Autodesk Inventor part; units mm, degrees
(part 2 of 2)
sketch "Boceto13" plane through (0, 0, 0) normal (0, 0, -1) x (-1, 0, 0)
  circle A0 centre (-56.75, 72.0206) radius 8 projected
  line L0 (-56.75, 72.0206) -> (-80.75, 72.0206)
  line L1 (-80.75, 105.95) -> (-80.75, -105.95) projected
  line L2 (-80.75, 72.0206) -> (80.75, 72.0206)
  line L3 (80.75, -105.95) -> (80.75, 105.95) projected
  circle A1 centre (-56.75, 43.1636) radius 8 projected
  line L4 (-56.75, 43.1636) -> (-56.75, 72.0206)
  line L5 (-56.75, 43.1636) -> (-80.75, 43.1636)
  line L6 (-80.75, 43.1636) -> (80.75, 43.1636)
  line L7 (-56.75, 14.3066) -> (-56.75, 43.1636)
  line L8 (-56.75, 14.3066) -> (-80.75, 14.3066)
  line L9 (-80.75, 14.3066) -> (80.75, 14.3066)
  line L10 (-56.75, -14.5504) -> (-56.75, 14.3066)
  line L11 (-56.75, -14.5504) -> (-80.75, -14.5504)
  line L12 (-80.75, -14.5504) -> (80.75, -14.5504)
  line L13 (-56.75, -43.4074) -> (-56.75, -14.5504)
  line L14 (-56.75, -43.4074) -> (-80.75, -43.4074)
  line L15 (-80.75, -43.4074) -> (80.75, -43.4074)
  line L16 (-56.75, -72.2644) -> (-56.75, -43.4074)
  line L17 (-56.75, -98.6167) -> (-56.75, -69.7597)
  line L18 (-56.75, -72.2644) -> (-80.75, -72.2644)
  line L19 (-80.75, -72.2644) -> (80.75, -72.2644)
  line L20 (-56.75, -101.1214) -> (-56.75, -72.2644)
  line L21 (43.5, 62.1456) -> (30.5, 62.1456) projected
  line L22 (30.5, 62.1456) -> (-80.75, 62.1456)
  line L23 (30.5, 81.8956) -> (43.5, 81.8956) projected
  line L24 (30.5, 81.8956) -> (80.75, 81.8956)
  line L25 (30.5, 62.1456) -> (80.75, 62.1456)
  line L26 (30.5, 81.8956) -> (-80.75, 81.8956)
  line L27 (30.5, 33.2886) -> (-80.75, 33.2886)
  line L28 (30.5, 53.0386) -> (80.75, 53.0386)
  line L29 (30.5, 33.2886) -> (80.75, 33.2886)
  line L30 (30.5, 53.0386) -> (-80.75, 53.0386)
  line L31 (30.5, 4.4316) -> (-80.75, 4.4316)
  line L32 (30.5, 24.1816) -> (80.75, 24.1816)
  line L33 (30.5, 4.4316) -> (80.75, 4.4316)
  line L34 (30.5, 24.1816) -> (-80.75, 24.1816)
  line L35 (30.5, -24.4254) -> (-80.75, -24.4254)
  line L36 (30.5, -4.6754) -> (80.75, -4.6754)
  line L37 (30.5, -24.4254) -> (80.75, -24.4254)
  line L38 (30.5, -4.6754) -> (-80.75, -4.6754)
  line L39 (30.5, -53.2824) -> (-80.75, -53.2824)
  line L40 (30.5, -33.5324) -> (80.75, -33.5324)
  line L41 (30.5, -53.2824) -> (80.75, -53.2824)
  line L42 (30.5, -33.5324) -> (-80.75, -33.5324)
  line L43 (30.5, -82.1394) -> (-80.75, -82.1394)
  line L44 (30.5, -62.3894) -> (80.75, -62.3894)
  line L45 (30.5, -82.1394) -> (80.75, -82.1394)
  line L46 (30.5, -62.3894) -> (-80.75, -62.3894)
  line L47 (-80.6263, 81.8524) -> (-64.7122, 81.8524) construction
  line L48 (-64.7122, 81.8524) -> (-64.7122, 62.1807) construction
  line L49 (-64.7122, 62.1807) -> (-80.6263, 62.1807) construction
  line L50 (-80.6263, 62.1807) -> (-80.6263, 81.8524) construction
  line L51 (-83, 108.2) -> (83, 108.2) projected
  line L52 (0, 108.2) -> (0, -109.1206)
  line L53 (-80.6263, 52.9954) -> (-64.7122, 52.9954) construction
  line L54 (-64.7122, 52.9954) -> (-64.7122, 33.3237) construction
  line L55 (-64.7122, 33.3237) -> (-80.6263, 33.3237) construction
  line L56 (-80.6263, 33.3237) -> (-80.6263, 52.9954) construction
  line L57 (-80.6263, 24.1384) -> (-64.7122, 24.1384) construction
  line L58 (-64.7122, 24.1384) -> (-64.7122, 4.4667) construction
  line L59 (-64.7122, 4.4667) -> (-80.6263, 4.4667) construction
  line L60 (-80.6263, 4.4667) -> (-80.6263, 24.1384) construction
  line L61 (-80.6263, -4.7186) -> (-64.7122, -4.7186) construction
  line L62 (-64.7122, -4.7186) -> (-64.7122, -24.3903) construction
  line L63 (-64.7122, -24.3903) -> (-80.6263, -24.3903) construction
  line L64 (-80.6263, -24.3903) -> (-80.6263, -4.7186) construction
  line L65 (-80.6263, -33.5756) -> (-64.7122, -33.5756) construction
  line L66 (-64.7122, -33.5756) -> (-64.7122, -53.2473) construction
  line L67 (-64.7122, -53.2473) -> (-80.6263, -53.2473) construction
  line L68 (-80.6263, -53.2473) -> (-80.6263, -33.5756) construction
  line L69 (-80.6263, -62.4326) -> (-64.7122, -62.4326) construction
  line L70 (-64.7122, -62.4326) -> (-64.7122, -82.1043) construction
  line L71 (-64.7122, -82.1043) -> (-80.6263, -82.1043) construction
  line L72 (-80.6263, -82.1043) -> (-80.6263, -62.4326) construction
  line L73 (-72.6693, 72.0206) -> (-88.5883, 72.0206)
  circle A2 centre (56.75, 72.0206) radius 8 projected
  circle A3 centre (56.75, -72.2644) radius 8 projected
  line L74 (56.75, 72.0206) -> (56.75, -72.2644)
  line L75 (64.7119, 81.8524) -> (80.6261, 81.8524) construction
  line L76 (80.6261, 81.8524) -> (80.6261, 62.1807) construction
  line L77 (80.6261, 62.1807) -> (64.7119, 62.1807) construction
  line L78 (64.7119, 62.1807) -> (64.7119, 81.8524) construction
  line L79 (56.75, 43.1636) -> (56.75, 14.3066)
  line L80 (56.75, -14.5504) -> (56.75, 14.3066)
  circle A4 centre (56.75, -43.4074) radius 8 projected
  line L81 (56.75, -72.2644) -> (56.75, -43.4074)
  line L82 (56.75, -43.4074) -> (56.75, -14.5504)
  line L83 (64.7119, 33.3237) -> (64.7119, 52.9954) construction
  line L84 (64.7119, 52.9954) -> (80.6261, 52.9954) construction
  line L85 (80.6261, 52.9954) -> (80.6261, 33.3237) construction
  line L86 (80.6261, 33.3237) -> (64.7119, 33.3237) construction
  line L87 (64.7119, 4.4667) -> (64.7119, 24.1384) construction
  line L88 (64.7119, 24.1384) -> (80.6261, 24.1384) construction
  line L89 (80.6261, 24.1384) -> (80.6261, 4.4667) construction
  line L90 (80.6261, 4.4667) -> (64.7119, 4.4667) construction
  line L91 (64.7119, -24.3903) -> (64.7119, -4.7186) construction
  line L92 (64.7119, -4.7186) -> (80.6261, -4.7186) construction
  line L93 (80.6261, -4.7186) -> (80.6261, -24.3903) construction
  line L94 (80.6261, -24.3903) -> (64.7119, -24.3903) construction
  line L95 (64.7119, -53.2473) -> (64.7119, -33.5756) construction
  line L96 (64.7119, -33.5756) -> (80.6261, -33.5756) construction
  line L97 (80.6261, -33.5756) -> (80.6261, -53.2473) construction
  line L98 (80.6261, -53.2473) -> (64.7119, -53.2473) construction
  line L99 (64.7119, -82.1043) -> (64.7119, -62.4326) construction
  line L100 (64.7119, -62.4326) -> (80.6261, -62.4326) construction
  line L101 (80.6261, -62.4326) -> (80.6261, -82.1043) construction
  line L102 (80.6261, -82.1043) -> (64.7119, -82.1043) construction
  spline S0 degree 2 poles (-73.0647, 70.8153) (-73.0647, 70.3655) (-73.3959, 69.629) (-73.7173, 69.3719) knots 0 0 0 1 2 2 2
  spline S1 degree 2 poles (-73.7173, 69.3719) (-74.0386, 69.1149) (-74.9135, 68.838) (-75.5413, 68.838) knots 0 0 0 1 2 2 2
  spline S2 degree 2 poles (-75.5413, 68.838) (-76.2532, 68.838) (-77.2715, 69.0753) (-77.5928, 69.2236) knots 0 0 0 1 2 2 2
  line L103 (-77.5928, 69.2236) -> (-77.5928, 70.5484)
  line L104 (-77.5928, 70.5484) -> (-77.4445, 70.5484)
  spline S3 degree 2 poles (-77.4445, 70.5484) (-77.1083, 70.3358) (-76.2037, 70.0195) (-75.828, 70.0195) knots 0 0 0 1 2 2 2
  spline S4 degree 2 poles (-75.828, 70.0195) (-75.6056, 70.0195) (-75.0865, 70.0986) (-74.9086, 70.2271) knots 0 0 0 1 2 2 2
  spline S5 degree 2 poles (-74.9086, 70.2271) (-74.7702, 70.3309) (-74.6021, 70.6324) (-74.6021, 70.9043) knots 0 0 0 1 2 2 2
  spline S6 degree 2 poles (-74.6021, 70.9043) (-74.6021, 71.1762) (-74.8394, 71.4679) (-75.0371, 71.5371) knots 0 0 0 1 2 2 2
  spline S7 degree 2 poles (-75.0371, 71.5371) (-75.2348, 71.6063) (-75.7835, 71.6211) (-75.9961, 71.6211) knots 0 0 0 1 2 2 2
  line L105 (-75.9961, 71.6211) -> (-76.2581, 71.6211)
  line L106 (-76.2581, 71.6211) -> (-76.2581, 72.6938)
  line L107 (-76.2581, 72.6938) -> (-76.0159, 72.6938)
  spline S8 degree 2 poles (-76.0159, 72.6938) (-75.7391, 72.6938) (-75.2694, 72.7432) (-75.1063, 72.8174) knots 0 0 0 1 2 2 2
  spline S9 degree 2 poles (-75.1063, 72.8174) (-74.9432, 72.8965) (-74.7603, 73.1733) (-74.7603, 73.4106) knots 0 0 0 1 2 2 2
  spline S10 degree 2 poles (-74.7603, 73.4106) (-74.7603, 73.5984) (-74.9333, 73.8307) (-75.0569, 73.895) knots 0 0 0 1 2 2 2
  spline S11 degree 2 poles (-75.0569, 73.895) (-75.2052, 73.9691) (-75.6006, 74.0186) (-75.7391, 74.0186) knots 0 0 0 1 2 2 2
  spline S12 degree 2 poles (-75.7391, 74.0186) (-75.9615, 74.0186) (-76.4311, 73.9148) (-76.6486, 73.8307) knots 0 0 0 1 2 2 2
  spline S13 degree 2 poles (-76.6486, 73.8307) (-76.8216, 73.7665) (-77.1973, 73.5589) (-77.2863, 73.5045) knots 0 0 0 1 2 2 2
  line L108 (-77.2863, 73.5045) -> (-77.4148, 73.5045)
  line L109 (-77.4148, 73.5045) -> (-77.4148, 74.8095)
  spline S14 degree 2 poles (-77.4148, 74.8095) (-77.0985, 74.943) (-76.0307, 75.1951) (-75.4721, 75.1951) knots 0 0 0 1 2 2 2
  spline S15 degree 2 poles (-75.4721, 75.1951) (-74.9284, 75.1951) (-74.1275, 75.0072) (-73.8458, 74.8243) knots 0 0 0 1 2 2 2
  spline S16 degree 2 poles (-73.8458, 74.8243) (-73.5344, 74.6315) (-73.2229, 74.0384) (-73.2229, 73.6676) knots 0 0 0 1 2 2 2
  spline S17 degree 2 poles (-73.2229, 73.6676) (-73.2229, 73.1436) (-73.826, 72.3626) (-74.3203, 72.2489) knots 0 0 0 1 2 2 2
  line L110 (-74.3203, 72.2489) -> (-74.3203, 72.1896)
  spline S18 degree 2 poles (-74.3203, 72.1896) (-74.1028, 72.1599) (-73.6876, 72.0017) (-73.4899, 71.8238) knots 0 0 0 1 2 2 2
  spline S19 degree 2 poles (-73.4899, 71.8238) (-73.307, 71.6656) (-73.0647, 71.1614) (-73.0647, 70.8153) knots 0 0 0 1 2 2 2
  line L111 (-67.7013, 73.8555) -> (-70.3064, 68.9666)
  line L112 (-70.3064, 68.9666) -> (-72.0069, 68.9666)
  line L113 (-72.0069, 68.9666) -> (-69.2831, 73.9148)
  line L114 (-69.2831, 73.9148) -> (-72.1898, 73.9148)
  line L115 (-72.1898, 73.9148) -> (-72.1898, 75.0666)
  line L116 (-72.1898, 75.0666) -> (-67.7013, 75.0666)
  line L117 (-67.7013, 75.0666) -> (-67.7013, 73.8555)
  spline S20 degree 2 poles (-73.0647, 41.9608) (-73.0647, 41.511) (-73.3959, 40.7744) (-73.7173, 40.5174) knots 0 0 0 1 2 2 2
  spline S21 degree 2 poles (-73.7173, 40.5174) (-74.0386, 40.2603) (-74.9135, 39.9835) (-75.5413, 39.9835) knots 0 0 0 1 2 2 2
  spline S22 degree 2 poles (-75.5413, 39.9835) (-76.2532, 39.9835) (-77.2715, 40.2208) (-77.5928, 40.3691) knots 0 0 0 1 2 2 2
  line L118 (-77.5928, 40.3691) -> (-77.5928, 41.6939)
  line L119 (-77.5928, 41.6939) -> (-77.4445, 41.6939)
  spline S23 degree 2 poles (-77.4445, 41.6939) (-77.1083, 41.4813) (-76.2037, 41.1649) (-75.828, 41.1649) knots 0 0 0 1 2 2 2
  spline S24 degree 2 poles (-75.828, 41.1649) (-75.6056, 41.1649) (-75.0865, 41.244) (-74.9086, 41.3726) knots 0 0 0 1 2 2 2
  spline S25 degree 2 poles (-74.9086, 41.3726) (-74.7702, 41.4764) (-74.6021, 41.7779) (-74.6021, 42.0498) knots 0 0 0 1 2 2 2
  spline S26 degree 2 poles (-74.6021, 42.0498) (-74.6021, 42.3217) (-74.8394, 42.6133) (-75.0371, 42.6825) knots 0 0 0 1 2 2 2
  spline S27 degree 2 poles (-75.0371, 42.6825) (-75.2348, 42.7517) (-75.7835, 42.7666) (-75.9961, 42.7666) knots 0 0 0 1 2 2 2
  line L120 (-75.9961, 42.7666) -> (-76.2581, 42.7666)
  line L121 (-76.2581, 42.7666) -> (-76.2581, 43.8393)
  line L122 (-76.2581, 43.8393) -> (-76.0159, 43.8393)
  spline S28 degree 2 poles (-76.0159, 43.8393) (-75.7391, 43.8393) (-75.2694, 43.8887) (-75.1063, 43.9628) knots 0 0 0 1 2 2 2
  spline S29 degree 2 poles (-75.1063, 43.9628) (-74.9432, 44.0419) (-74.7603, 44.3188) (-74.7603, 44.556) knots 0 0 0 1 2 2 2
  spline S30 degree 2 poles (-74.7603, 44.556) (-74.7603, 44.7439) (-74.9333, 44.9762) (-75.0569, 45.0405) knots 0 0 0 1 2 2 2
  spline S31 degree 2 poles (-75.0569, 45.0405) (-75.2052, 45.1146) (-75.6006, 45.1641) (-75.7391, 45.1641) knots 0 0 0 1 2 2 2
  spline S32 degree 2 poles (-75.7391, 45.1641) (-75.9615, 45.1641) (-76.4311, 45.0602) (-76.6486, 44.9762) knots 0 0 0 1 2 2 2
  spline S33 degree 2 poles (-76.6486, 44.9762) (-76.8216, 44.9119) (-77.1973, 44.7043) (-77.2863, 44.65) knots 0 0 0 1 2 2 2
  line L123 (-77.2863, 44.65) -> (-77.4148, 44.65)
  line L124 (-77.4148, 44.65) -> (-77.4148, 45.955)
  spline S34 degree 2 poles (-77.4148, 45.955) (-77.0985, 46.0884) (-76.0307, 46.3406) (-75.4721, 46.3406) knots 0 0 0 1 2 2 2
  spline S35 degree 2 poles (-75.4721, 46.3406) (-74.9284, 46.3406) (-74.1275, 46.1527) (-73.8458, 45.9698) knots 0 0 0 1 2 2 2
  spline S36 degree 2 poles (-73.8458, 45.9698) (-73.5344, 45.777) (-73.2229, 45.1838) (-73.2229, 44.8131) knots 0 0 0 1 2 2 2
  spline S37 degree 2 poles (-73.2229, 44.8131) (-73.2229, 44.2891) (-73.826, 43.5081) (-74.3203, 43.3944) knots 0 0 0 1 2 2 2
  line L125 (-74.3203, 43.3944) -> (-74.3203, 43.335)
  spline S38 degree 2 poles (-74.3203, 43.335) (-74.1028, 43.3054) (-73.6876, 43.1472) (-73.4899, 42.9692) knots 0 0 0 1 2 2 2
  spline S39 degree 2 poles (-73.4899, 42.9692) (-73.307, 42.8111) (-73.0647, 42.3068) (-73.0647, 41.9608) knots 0 0 0 1 2 2 2
  spline S40 degree 2 poles (-67.5827, 41.8076) (-67.5827, 41.4171) (-67.9089, 40.7398) (-68.2203, 40.4927) knots 0 0 0 1 2 2 2
  spline S41 degree 2 poles (-68.2203, 40.4927) (-68.5318, 40.2455) (-69.4265, 39.9687) (-70.0049, 39.9687) knots 0 0 0 1 2 2 2
  spline S42 degree 2 poles (-70.0049, 39.9687) (-70.6228, 39.9687) (-71.5472, 40.2504) (-71.8438, 40.4927) knots 0 0 0 1 2 2 2
  spline S43 degree 2 poles (-71.8438, 40.4927) (-72.1354, 40.7349) (-72.4122, 41.3923) (-72.4122, 41.7581) knots 0 0 0 1 2 2 2
  spline S44 degree 2 poles (-72.4122, 41.7581) (-72.4122, 42.2821) (-71.8339, 42.9791) (-71.2852, 43.2115) knots 0 0 0 1 2 2 2
  line L126 (-71.2852, 43.2115) -> (-71.2852, 43.2362)
  spline S45 degree 2 poles (-71.2852, 43.2362) (-71.824, 43.4982) (-72.2491, 44.2446) (-72.2491, 44.7043) knots 0 0 0 1 2 2 2
  spline S46 degree 2 poles (-72.2491, 44.7043) (-72.2491, 45.0405) (-71.9525, 45.6287) (-71.6609, 45.8611) knots 0 0 0 1 2 2 2
  spline S47 degree 2 poles (-71.6609, 45.8611) (-71.3791, 46.0835) (-70.5239, 46.3504) (-69.99, 46.3504) knots 0 0 0 1 2 2 2
  spline S48 degree 2 poles (-69.99, 46.3504) (-69.4265, 46.3504) (-68.5861, 46.1082) (-68.3143, 45.9105) knots 0 0 0 1 2 2 2
  spline S49 degree 2 poles (-68.3143, 45.9105) (-68.0374, 45.7128) (-67.7408, 45.1393) (-67.7408, 44.8081) knots 0 0 0 1 2 2 2
  spline S50 degree 2 poles (-67.7408, 44.8081) (-67.7408, 44.3731) (-68.245, 43.6761) (-68.7641, 43.4339) knots 0 0 0 1 2 2 2
  line L127 (-68.7641, 43.4339) -> (-68.7641, 43.4141)
  spline S51 degree 2 poles (-68.7641, 43.4141) (-68.1561, 43.167) (-67.5827, 42.3662) (-67.5827, 41.8076) knots 0 0 0 1 2 2 2
  spline S52 degree 2 poles (-69.0953, 41.7433) (-69.0953, 42.0448) (-69.3523, 42.3612) (-69.7676, 42.5639) knots 0 0 0 1 2 2 2
  spline S53 degree 2 poles (-69.7676, 42.5639) (-69.8862, 42.6183) (-70.3361, 42.7913) (-70.5091, 42.8654) knots 0 0 0 1 2 2 2
  spline S54 degree 2 poles (-70.5091, 42.8654) (-70.6673, 42.7072) (-70.9194, 42.2327) (-70.9194, 41.9509) knots 0 0 0 1 2 2 2
  spline S55 degree 2 poles (-70.9194, 41.9509) (-70.9194, 41.5258) (-70.3756, 41.0166) (-69.9356, 41.0166) knots 0 0 0 1 2 2 2
  spline S56 degree 2 poles (-69.9356, 41.0166) (-69.8121, 41.0166) (-69.5056, 41.0957) (-69.3869, 41.1748) knots 0 0 0 1 2 2 2
  spline S57 degree 2 poles (-69.3869, 41.1748) (-69.2535, 41.2688) (-69.0953, 41.5258) (-69.0953, 41.7433) knots 0 0 0 1 2 2 2
  spline S58 degree 2 poles (-69.2288, 44.6302) (-69.2288, 44.9416) (-69.6391, 45.3124) (-69.99, 45.3124) knots 0 0 0 1 2 2 2
  spline S59 degree 2 poles (-69.99, 45.3124) (-70.3262, 45.3124) (-70.7365, 44.9762) (-70.7365, 44.729) knots 0 0 0 1 2 2 2
  spline S60 degree 2 poles (-70.7365, 44.729) (-70.7365, 44.4868) (-70.4893, 44.1853) (-70.2273, 44.0617) knots 0 0 0 1 2 2 2
  spline S61 degree 2 poles (-70.2273, 44.0617) (-70.1136, 44.0024) (-69.7972, 43.8788) (-69.5352, 43.7799) knots 0 0 0 1 2 2 2
  spline S62 degree 2 poles (-69.5352, 43.7799) (-69.3771, 43.9876) (-69.2288, 44.3781) (-69.2288, 44.6302) knots 0 0 0 1 2 2 2
  spline S63 degree 2 poles (-73.0647, 13.1013) (-73.0647, 12.6515) (-73.3959, 11.915) (-73.7173, 11.6579) knots 0 0 0 1 2 2 2
  spline S64 degree 2 poles (-73.7173, 11.6579) (-74.0386, 11.4009) (-74.9135, 11.124) (-75.5413, 11.124) knots 0 0 0 1 2 2 2
  spline S65 degree 2 poles (-75.5413, 11.124) (-76.2532, 11.124) (-77.2715, 11.3613) (-77.5928, 11.5096) knots 0 0 0 1 2 2 2
  line L128 (-77.5928, 11.5096) -> (-77.5928, 12.8344)
  line L129 (-77.5928, 12.8344) -> (-77.4445, 12.8344)
  spline S66 degree 2 poles (-77.4445, 12.8344) (-77.1083, 12.6218) (-76.2037, 12.3055) (-75.828, 12.3055) knots 0 0 0 1 2 2 2
  spline S67 degree 2 poles (-75.828, 12.3055) (-75.6056, 12.3055) (-75.0865, 12.3846) (-74.9086, 12.5131) knots 0 0 0 1 2 2 2
  spline S68 degree 2 poles (-74.9086, 12.5131) (-74.7702, 12.6169) (-74.6021, 12.9184) (-74.6021, 13.1903) knots 0 0 0 1 2 2 2
  spline S69 degree 2 poles (-74.6021, 13.1903) (-74.6021, 13.4622) (-74.8394, 13.7539) (-75.0371, 13.8231) knots 0 0 0 1 2 2 2
  spline S70 degree 2 poles (-75.0371, 13.8231) (-75.2348, 13.8923) (-75.7835, 13.9071) (-75.9961, 13.9071) knots 0 0 0 1 2 2 2
  line L130 (-75.9961, 13.9071) -> (-76.2581, 13.9071)
  line L131 (-76.2581, 13.9071) -> (-76.2581, 14.9798)
  line L132 (-76.2581, 14.9798) -> (-76.0159, 14.9798)
  spline S71 degree 2 poles (-76.0159, 14.9798) (-75.7391, 14.9798) (-75.2694, 15.0292) (-75.1063, 15.1034) knots 0 0 0 1 2 2 2
  spline S72 degree 2 poles (-75.1063, 15.1034) (-74.9432, 15.1825) (-74.7603, 15.4593) (-74.7603, 15.6966) knots 0 0 0 1 2 2 2
  spline S73 degree 2 poles (-74.7603, 15.6966) (-74.7603, 15.8844) (-74.9333, 16.1167) (-75.0569, 16.181) knots 0 0 0 1 2 2 2
  spline S74 degree 2 poles (-75.0569, 16.181) (-75.2052, 16.2551) (-75.6006, 16.3046) (-75.7391, 16.3046) knots 0 0 0 1 2 2 2
  spline S75 degree 2 poles (-75.7391, 16.3046) (-75.9615, 16.3046) (-76.4311, 16.2008) (-76.6486, 16.1167) knots 0 0 0 1 2 2 2
  spline S76 degree 2 poles (-76.6486, 16.1167) (-76.8216, 16.0525) (-77.1973, 15.8449) (-77.2863, 15.7905) knots 0 0 0 1 2 2 2
  line L133 (-77.2863, 15.7905) -> (-77.4148, 15.7905)
  line L134 (-77.4148, 15.7905) -> (-77.4148, 17.0955)
  spline S77 degree 2 poles (-77.4148, 17.0955) (-77.0985, 17.229) (-76.0307, 17.4811) (-75.4721, 17.4811) knots 0 0 0 1 2 2 2
  spline S78 degree 2 poles (-75.4721, 17.4811) (-74.9284, 17.4811) (-74.1275, 17.2932) (-73.8458, 17.1103) knots 0 0 0 1 2 2 2
  spline S79 degree 2 poles (-73.8458, 17.1103) (-73.5344, 16.9175) (-73.2229, 16.3244) (-73.2229, 15.9536) knots 0 0 0 1 2 2 2
  spline S80 degree 2 poles (-73.2229, 15.9536) (-73.2229, 15.4296) (-73.826, 14.6486) (-74.3203, 14.5349) knots 0 0 0 1 2 2 2
  line L135 (-74.3203, 14.5349) -> (-74.3203, 14.4756)
  spline S81 degree 2 poles (-74.3203, 14.4756) (-74.1028, 14.4459) (-73.6876, 14.2877) (-73.4899, 14.1098) knots 0 0 0 1 2 2 2
  spline S82 degree 2 poles (-73.4899, 14.1098) (-73.307, 13.9516) (-73.0647, 13.4474) (-73.0647, 13.1013) knots 0 0 0 1 2 2 2
  spline S83 degree 2 poles (-67.726, 14.6436) (-67.726, 13.8675) (-68.0869, 12.5724) (-68.4675, 12.1077) knots 0 0 0 1 2 2 2
  spline S84 degree 2 poles (-68.4675, 12.1077) (-68.863, 11.6381) (-70.0296, 11.1339) (-70.8798, 11.1339) knots 0 0 0 1 2 2 2
  spline S85 degree 2 poles (-70.8798, 11.1339) (-71.1665, 11.1339) (-71.7894, 11.2081) (-71.8932, 11.2377) knots 0 0 0 1 2 2 2
  line L136 (-71.8932, 11.2377) -> (-71.8932, 12.434)
  line L137 (-71.8932, 12.434) -> (-71.7745, 12.434)
  spline S86 degree 2 poles (-71.7745, 12.434) (-71.6609, 12.3747) (-71.2357, 12.2462) (-70.865, 12.2462) knots 0 0 0 1 2 2 2
  spline S87 degree 2 poles (-70.865, 12.2462) (-70.5634, 12.2462) (-70.0049, 12.4043) (-69.8071, 12.5774) knots 0 0 0 1 2 2 2
  spline S88 degree 2 poles (-69.8071, 12.5774) (-69.5946, 12.7603) (-69.3177, 13.2991) (-69.2683, 13.7044) knots 0 0 0 1 2 2 2
  spline S89 degree 2 poles (-69.2683, 13.7044) (-69.5946, 13.5017) (-70.1581, 13.2842) (-70.5783, 13.2842) knots 0 0 0 1 2 2 2
  spline S90 degree 2 poles (-70.5783, 13.2842) (-70.8897, 13.2842) (-71.4681, 13.4523) (-71.7053, 13.6303) knots 0 0 0 1 2 2 2
  spline S91 degree 2 poles (-71.7053, 13.6303) (-72.0217, 13.8725) (-72.3925, 14.6486) (-72.3925, 15.2616) knots 0 0 0 1 2 2 2
  spline S92 degree 2 poles (-72.3925, 15.2616) (-72.3925, 15.741) (-72.0662, 16.5468) (-71.7696, 16.8434) knots 0 0 0 1 2 2 2
  spline S93 degree 2 poles (-71.7696, 16.8434) (-71.473, 17.14) (-70.6129, 17.4761) (-70.0839, 17.4761) knots 0 0 0 1 2 2 2
  spline S94 degree 2 poles (-70.0839, 17.4761) (-69.5501, 17.4761) (-68.7245, 17.1795) (-68.428, 16.8681) knots 0 0 0 1 2 2 2
  spline S95 degree 2 poles (-68.428, 16.8681) (-68.0819, 16.5221) (-67.726, 15.4247) (-67.726, 14.6436) knots 0 0 0 1 2 2 2
  spline S96 degree 2 poles (-69.2436, 14.871) (-69.2436, 15.3703) (-69.4117, 16.0129) (-69.5649, 16.1909) knots 0 0 0 1 2 2 2
  spline S97 degree 2 poles (-69.5649, 16.1909) (-69.6687, 16.3244) (-69.9356, 16.4381) (-70.0889, 16.4381) knots 0 0 0 1 2 2 2
  spline S98 degree 2 poles (-70.0889, 16.4381) (-70.2273, 16.4381) (-70.4844, 16.3293) (-70.603, 16.1909) knots 0 0 0 1 2 2 2
  spline S99 degree 2 poles (-70.603, 16.1909) (-70.7068, 16.0722) (-70.8551, 15.6125) (-70.8551, 15.3406) knots 0 0 0 1 2 2 2
  spline S100 degree 2 poles (-70.8551, 15.3406) (-70.8551, 15.044) (-70.7019, 14.6634) (-70.5733, 14.5497) knots 0 0 0 1 2 2 2
  spline S101 degree 2 poles (-70.5733, 14.5497) (-70.4399, 14.436) (-70.1087, 14.347) (-69.901, 14.347) knots 0 0 0 1 2 2 2
  spline S102 degree 2 poles (-69.901, 14.347) (-69.728, 14.347) (-69.3672, 14.441) (-69.2535, 14.4904) knots 0 0 0 1 2 2 2
  spline S103 degree 2 poles (-69.2535, 14.4904) (-69.2535, 14.5349) (-69.2436, 14.703) (-69.2436, 14.871) knots 0 0 0 1 2 2 2
  line L138 (-72.8374, -16.1783) -> (-73.6629, -16.1783)
  line L139 (-73.6629, -16.1783) -> (-73.6629, -17.6168)
  line L140 (-73.6629, -17.6168) -> (-75.1409, -17.6168)
  line L141 (-75.1409, -17.6168) -> (-75.1409, -16.1783)
  line L142 (-75.1409, -16.1783) -> (-77.8301, -16.1783)
  line L143 (-77.8301, -16.1783) -> (-77.8301, -15.0414)
  line L144 (-77.8301, -15.0414) -> (-75.1903, -11.502)
  line L145 (-75.1903, -11.502) -> (-73.6629, -11.502)
  line L146 (-73.6629, -11.502) -> (-73.6629, -15.0809)
  line L147 (-73.6629, -15.0809) -> (-72.8374, -15.0809)
  line L148 (-72.8374, -15.0809) -> (-72.8374, -16.1783)
  line L149 (-75.1409, -15.0809) -> (-75.1409, -13.0047)
  line L150 (-75.1409, -13.0047) -> (-76.6882, -15.0809)
  line L151 (-76.6882, -15.0809) -> (-75.1409, -15.0809)
  spline S104 degree 2 poles (-67.6469, -14.552) (-67.6469, -15.3429) (-67.899, -16.5293) (-68.1808, -16.9297) knots 0 0 0 1 2 2 2
  spline S105 degree 2 poles (-68.1808, -16.9297) (-68.4576, -17.3251) (-69.3523, -17.7305) (-69.995, -17.7305) knots 0 0 0 1 2 2 2
  spline S106 degree 2 poles (-69.995, -17.7305) (-70.6425, -17.7305) (-71.5323, -17.3251) (-71.8141, -16.9198) knots 0 0 0 1 2 2 2
  spline S107 degree 2 poles (-71.8141, -16.9198) (-72.0959, -16.5194) (-72.348, -15.3429) (-72.348, -14.552) knots 0 0 0 1 2 2 2
  spline S108 degree 2 poles (-72.348, -14.552) (-72.348, -13.7413) (-72.0959, -12.5944) (-71.8092, -12.1792) knots 0 0 0 1 2 2 2
  spline S109 degree 2 poles (-71.8092, -12.1792) (-71.5224, -11.7739) (-70.6178, -11.3784) (-69.995, -11.3784) knots 0 0 0 1 2 2 2
  spline S110 degree 2 poles (-69.995, -11.3784) (-69.3375, -11.3784) (-68.4576, -11.7936) (-68.1758, -12.2039) knots 0 0 0 1 2 2 2
  spline S111 degree 2 poles (-68.1758, -12.2039) (-67.899, -12.6043) (-67.6469, -13.7858) (-67.6469, -14.552) knots 0 0 0 1 2 2 2
  spline S112 degree 2 poles (-69.1843, -14.552) (-69.1843, -13.42) (-69.555, -12.5055) (-69.995, -12.5055) knots 0 0 0 1 2 2 2
  spline S113 degree 2 poles (-69.995, -12.5055) (-70.4349, -12.5055) (-70.8106, -13.42) (-70.8106, -14.5569) knots 0 0 0 1 2 2 2
  spline S114 degree 2 poles (-70.8106, -14.5569) (-70.8106, -15.6741) (-70.4349, -16.6034) (-69.995, -16.6034) knots 0 0 0 1 2 2 2
  spline S115 degree 2 poles (-69.995, -16.6034) (-69.56, -16.6034) (-69.1843, -15.6741) (-69.1843, -14.552) knots 0 0 0 1 2 2 2
  line L152 (-72.8374, -45.0378) -> (-73.6629, -45.0378)
  line L153 (-73.6629, -45.0378) -> (-73.6629, -46.4763)
  line L154 (-73.6629, -46.4763) -> (-75.1409, -46.4763)
  line L155 (-75.1409, -46.4763) -> (-75.1409, -45.0378)
  line L156 (-75.1409, -45.0378) -> (-77.8301, -45.0378)
  line L157 (-77.8301, -45.0378) -> (-77.8301, -43.9008)
  line L158 (-77.8301, -43.9008) -> (-75.1903, -40.3614)
  line L159 (-75.1903, -40.3614) -> (-73.6629, -40.3614)
  line L160 (-73.6629, -40.3614) -> (-73.6629, -43.9404)
  line L161 (-73.6629, -43.9404) -> (-72.8374, -43.9404)
  line L162 (-72.8374, -43.9404) -> (-72.8374, -45.0378)
  line L163 (-75.1409, -43.9404) -> (-75.1409, -41.8642)
  line L164 (-75.1409, -41.8642) -> (-76.6882, -43.9404)
  line L165 (-76.6882, -43.9404) -> (-75.1409, -43.9404)
  line L166 (-67.8397, -46.4614) -> (-71.8685, -46.4614)
  line L167 (-71.8685, -46.4614) -> (-71.8685, -45.3986)
  line L168 (-71.8685, -45.3986) -> (-70.5832, -45.3986)
  line L169 (-70.5832, -45.3986) -> (-70.5832, -42.1707)
  line L170 (-70.5832, -42.1707) -> (-71.8685, -42.1707)
  line L171 (-71.8685, -42.1707) -> (-71.8685, -41.1771)
  spline S116 degree 2 poles (-71.8685, -41.1771) (-71.5867, -41.1771) (-71.0281, -41.1029) (-70.86, -41.0238) knots 0 0 0 1 2 2 2
  spline S117 degree 2 poles (-70.86, -41.0238) (-70.6673, -40.925) (-70.4498, -40.5938) (-70.43, -40.3466) knots 0 0 0 1 2 2 2
  line L172 (-70.43, -40.3466) -> (-69.0953, -40.3466)
  line L173 (-69.0953, -40.3466) -> (-69.0953, -45.3986)
  line L174 (-69.0953, -45.3986) -> (-67.8397, -45.3986)
  line L175 (-67.8397, -45.3986) -> (-67.8397, -46.4614)
  line L176 (-72.8374, -73.9467) -> (-73.6629, -73.9467)
  line L177 (-73.6629, -73.9467) -> (-73.6629, -75.3852)
  line L178 (-73.6629, -75.3852) -> (-75.1409, -75.3852)
  line L179 (-75.1409, -75.3852) -> (-75.1409, -73.9467)
  line L180 (-75.1409, -73.9467) -> (-77.8301, -73.9467)
  line L181 (-77.8301, -73.9467) -> (-77.8301, -72.8097)
  line L182 (-77.8301, -72.8097) -> (-75.1903, -69.2703)
  line L183 (-75.1903, -69.2703) -> (-73.6629, -69.2703)
  line L184 (-73.6629, -69.2703) -> (-73.6629, -72.8493)
  line L185 (-73.6629, -72.8493) -> (-72.8374, -72.8493)
  line L186 (-72.8374, -72.8493) -> (-72.8374, -73.9467)
  line L187 (-75.1409, -72.8493) -> (-75.1409, -70.7731)
  line L188 (-75.1409, -70.7731) -> (-76.6882, -72.8493)
  line L189 (-76.6882, -72.8493) -> (-75.1409, -72.8493)
  line L190 (-67.5678, -75.3703) -> (-72.0514, -75.3703)
  line L191 (-72.0514, -75.3703) -> (-72.0514, -74.3767)
  spline S118 degree 2 poles (-72.0514, -74.3767) (-71.4829, -73.922) (-70.5733, -73.1212) (-70.2322, -72.7603) knots 0 0 0 1 2 2 2
  spline S119 degree 2 poles (-70.2322, -72.7603) (-69.7824, -72.2907) (-69.382, -71.5739) (-69.382, -71.1982) knots 0 0 0 1 2 2 2
  spline S120 degree 2 poles (-69.382, -71.1982) (-69.382, -70.7731) (-69.8912, -70.3183) (-70.3459, -70.3183) knots 0 0 0 1 2 2 2
  spline S121 degree 2 poles (-70.3459, -70.3183) (-70.5783, -70.3183) (-70.9935, -70.432) (-71.2061, -70.521) knots 0 0 0 1 2 2 2
  spline S122 degree 2 poles (-71.2061, -70.521) (-71.4137, -70.6149) (-71.7103, -70.8126) (-71.7844, -70.8621) knots 0 0 0 1 2 2 2
  line L192 (-71.7844, -70.8621) -> (-71.9031, -70.8621)
  line L193 (-71.9031, -70.8621) -> (-71.9031, -69.5323)
  spline S123 degree 2 poles (-71.9031, -69.5323) (-71.646, -69.4088) (-70.5486, -69.1517) (-70.0395, -69.1517) knots 0 0 0 1 2 2 2
  spline S124 degree 2 poles (-70.0395, -69.1517) (-68.9519, -69.1517) (-67.8348, -70.1206) (-67.8348, -70.9956) knots 0 0 0 1 2 2 2
  spline S125 degree 2 poles (-67.8348, -70.9956) (-67.8348, -71.5344) (-68.3439, -72.5725) (-68.9322, -73.1656) knots 0 0 0 1 2 2 2
  spline S126 degree 2 poles (-68.9322, -73.1656) (-69.3029, -73.5315) (-69.9999, -74.0999) (-70.1532, -74.2186) knots 0 0 0 1 2 2 2
  line L194 (-70.1532, -74.2186) -> (-67.5678, -74.2186)
  line L195 (-67.5678, -74.2186) -> (-67.5678, -75.3703)
  line L196 (72.5009, 70.3902) -> (71.6754, 70.3902)
  line L197 (71.6754, 70.3902) -> (71.6754, 68.9517)
  line L198 (71.6754, 68.9517) -> (70.1974, 68.9517)
  line L199 (70.1974, 68.9517) -> (70.1974, 70.3902)
  line L200 (70.1974, 70.3902) -> (67.5082, 70.3902)
  line L201 (67.5082, 70.3902) -> (67.5082, 71.5272)
  line L202 (67.5082, 71.5272) -> (70.1479, 75.0666)
  line L203 (70.1479, 75.0666) -> (71.6754, 75.0666)
  line L204 (71.6754, 75.0666) -> (71.6754, 71.4876)
  line L205 (71.6754, 71.4876) -> (72.5009, 71.4876)
  line L206 (72.5009, 71.4876) -> (72.5009, 70.3902)
  line L207 (70.1974, 71.4876) -> (70.1974, 73.5638)
  line L208 (70.1974, 73.5638) -> (68.6501, 71.4876)
  line L209 (68.6501, 71.4876) -> (70.1974, 71.4876)
  spline S127 degree 2 poles (77.6172, 70.8153) (77.6172, 70.3655) (77.286, 69.629) (76.9647, 69.3719) knots 0 0 0 1 2 2 2
  spline S128 degree 2 poles (76.9647, 69.3719) (76.6434, 69.1149) (75.7684, 68.838) (75.1406, 68.838) knots 0 0 0 1 2 2 2
  spline S129 degree 2 poles (75.1406, 68.838) (74.4288, 68.838) (73.4105, 69.0753) (73.0892, 69.2236) knots 0 0 0 1 2 2 2
  line L210 (73.0892, 69.2236) -> (73.0892, 70.5484)
  line L211 (73.0892, 70.5484) -> (73.2375, 70.5484)
  spline S130 degree 2 poles (73.2375, 70.5484) (73.5736, 70.3358) (74.4782, 70.0195) (74.8539, 70.0195) knots 0 0 0 1 2 2 2
  spline S131 degree 2 poles (74.8539, 70.0195) (75.0764, 70.0195) (75.5954, 70.0986) (75.7734, 70.2271) knots 0 0 0 1 2 2 2
  spline S132 degree 2 poles (75.7734, 70.2271) (75.9118, 70.3309) (76.0799, 70.6324) (76.0799, 70.9043) knots 0 0 0 1 2 2 2
  spline S133 degree 2 poles (76.0799, 70.9043) (76.0799, 71.1762) (75.8426, 71.4679) (75.6449, 71.5371) knots 0 0 0 1 2 2 2
  spline S134 degree 2 poles (75.6449, 71.5371) (75.4471, 71.6063) (74.8984, 71.6211) (74.6859, 71.6211) knots 0 0 0 1 2 2 2
  line L212 (74.6859, 71.6211) -> (74.4239, 71.6211)
  line L213 (74.4239, 71.6211) -> (74.4239, 72.6938)
  line L214 (74.4239, 72.6938) -> (74.6661, 72.6938)
  spline S135 degree 2 poles (74.6661, 72.6938) (74.9429, 72.6938) (75.4125, 72.7432) (75.5756, 72.8174) knots 0 0 0 1 2 2 2
  spline S136 degree 2 poles (75.5756, 72.8174) (75.7388, 72.8965) (75.9217, 73.1733) (75.9217, 73.4106) knots 0 0 0 1 2 2 2
  spline S137 degree 2 poles (75.9217, 73.4106) (75.9217, 73.5984) (75.7487, 73.8307) (75.6251, 73.895) knots 0 0 0 1 2 2 2
  spline S138 degree 2 poles (75.6251, 73.895) (75.4768, 73.9691) (75.0813, 74.0186) (74.9429, 74.0186) knots 0 0 0 1 2 2 2
  spline S139 degree 2 poles (74.9429, 74.0186) (74.7205, 74.0186) (74.2508, 73.9148) (74.0333, 73.8307) knots 0 0 0 1 2 2 2
  spline S140 degree 2 poles (74.0333, 73.8307) (73.8603, 73.7665) (73.4846, 73.5589) (73.3957, 73.5045) knots 0 0 0 1 2 2 2
  line L215 (73.3957, 73.5045) -> (73.2671, 73.5045)
  line L216 (73.2671, 73.5045) -> (73.2671, 74.8095)
  spline S141 degree 2 poles (73.2671, 74.8095) (73.5835, 74.943) (74.6513, 75.1951) (75.2098, 75.1951) knots 0 0 0 1 2 2 2
  spline S142 degree 2 poles (75.2098, 75.1951) (75.7536, 75.1951) (76.5544, 75.0072) (76.8362, 74.8243) knots 0 0 0 1 2 2 2
  spline S143 degree 2 poles (76.8362, 74.8243) (77.1476, 74.6315) (77.459, 74.0384) (77.459, 73.6676) knots 0 0 0 1 2 2 2
  spline S144 degree 2 poles (77.459, 73.6676) (77.459, 73.1436) (76.856, 72.3626) (76.3616, 72.2489) knots 0 0 0 1 2 2 2
  line L217 (76.3616, 72.2489) -> (76.3616, 72.1896)
  spline S145 degree 2 poles (76.3616, 72.1896) (76.5791, 72.1599) (76.9944, 72.0017) (77.1921, 71.8238) knots 0 0 0 1 2 2 2
  spline S146 degree 2 poles (77.1921, 71.8238) (77.375, 71.6656) (77.6172, 71.1614) (77.6172, 70.8153) knots 0 0 0 1 2 2 2
  line L218 (72.5009, 41.5406) -> (71.6754, 41.5406)
  line L219 (71.6754, 41.5406) -> (71.6754, 40.1021)
  line L220 (71.6754, 40.1021) -> (70.1974, 40.1021)
  line L221 (70.1974, 40.1021) -> (70.1974, 41.5406)
  line L222 (70.1974, 41.5406) -> (67.5082, 41.5406)
  line L223 (67.5082, 41.5406) -> (67.5082, 42.6776)
  line L224 (67.5082, 42.6776) -> (70.1479, 46.217)
  line L225 (70.1479, 46.217) -> (71.6754, 46.217)
  line L226 (71.6754, 46.217) -> (71.6754, 42.638)
  line L227 (71.6754, 42.638) -> (72.5009, 42.638)
  line L228 (72.5009, 42.638) -> (72.5009, 41.5406)
  line L229 (70.1974, 42.638) -> (70.1974, 44.7142)
  line L230 (70.1974, 44.7142) -> (68.6501, 42.638)
  line L231 (68.6501, 42.638) -> (70.1974, 42.638)
  line L232 (77.8446, 41.5406) -> (77.0191, 41.5406)
  line L233 (77.0191, 41.5406) -> (77.0191, 40.1021)
  line L234 (77.0191, 40.1021) -> (75.541, 40.1021)
  line L235 (75.541, 40.1021) -> (75.541, 41.5406)
  line L236 (75.541, 41.5406) -> (72.8519, 41.5406)
  line L237 (72.8519, 41.5406) -> (72.8519, 42.6776)
  line L238 (72.8519, 42.6776) -> (75.4916, 46.217)
  line L239 (75.4916, 46.217) -> (77.0191, 46.217)
  line L240 (77.0191, 46.217) -> (77.0191, 42.638)
  line L241 (77.0191, 42.638) -> (77.8446, 42.638)
  line L242 (77.8446, 42.638) -> (77.8446, 41.5406)
  line L243 (75.541, 42.638) -> (75.541, 44.7142)
  line L244 (75.541, 44.7142) -> (73.9938, 42.638)
  line L245 (73.9938, 42.638) -> (75.541, 42.638)
  line L246 (72.5009, 12.7405) -> (71.6754, 12.7405)
  line L247 (71.6754, 12.7405) -> (71.6754, 11.302)
  line L248 (71.6754, 11.302) -> (70.1974, 11.302)
  line L249 (70.1974, 11.302) -> (70.1974, 12.7405)
  line L250 (70.1974, 12.7405) -> (67.5082, 12.7405)
  line L251 (67.5082, 12.7405) -> (67.5082, 13.8774)
  line L252 (67.5082, 13.8774) -> (70.1479, 17.4168)
  line L253 (70.1479, 17.4168) -> (71.6754, 17.4168)
  line L254 (71.6754, 17.4168) -> (71.6754, 13.8379)
  line L255 (71.6754, 13.8379) -> (72.5009, 13.8379)
  line L256 (72.5009, 13.8379) -> (72.5009, 12.7405)
  line L257 (70.1974, 13.8379) -> (70.1974, 15.9141)
  line L258 (70.1974, 15.9141) -> (68.6501, 13.8379)
  line L259 (68.6501, 13.8379) -> (70.1974, 13.8379)
  spline S147 degree 2 poles (77.632, 13.3831) (77.632, 12.9036) (77.3058, 12.0929) (76.9845, 11.8013) knots 0 0 0 1 2 2 2
  spline S148 degree 2 poles (76.9845, 11.8013) (76.6632, 11.5096) (75.7833, 11.1883) (75.1406, 11.1883) knots 0 0 0 1 2 2 2
  spline S149 degree 2 poles (75.1406, 11.1883) (74.4585, 11.1932) (73.4797, 11.4157) (73.1584, 11.559) knots 0 0 0 1 2 2 2
  line L260 (73.1584, 11.559) -> (73.1584, 12.8888)
  line L261 (73.1584, 12.8888) -> (73.2968, 12.8888)
  spline S150 degree 2 poles (73.2968, 12.8888) (73.4154, 12.8245) (73.7021, 12.6564) (73.9345, 12.5675) knots 0 0 0 1 2 2 2
  spline S151 degree 2 poles (73.9345, 12.5675) (74.152, 12.4834) (74.6018, 12.3697) (74.8737, 12.3697) knots 0 0 0 1 2 2 2
  spline S152 degree 2 poles (74.8737, 12.3697) (75.111, 12.3697) (75.6646, 12.4884) (75.8327, 12.6466) knots 0 0 0 1 2 2 2
  spline S153 degree 2 poles (75.8327, 12.6466) (75.9563, 12.7701) (76.0947, 13.0717) (76.0947, 13.3238) knots 0 0 0 1 2 2 2
  spline S154 degree 2 poles (76.0947, 13.3238) (76.0947, 13.5413) (75.9167, 13.8478) (75.7734, 13.9417) knots 0 0 0 1 2 2 2
  spline S155 degree 2 poles (75.7734, 13.9417) (75.5658, 14.0801) (74.9726, 14.1592) (74.76, 14.1592) knots 0 0 0 1 2 2 2
  spline S156 degree 2 poles (74.76, 14.1592) (74.4239, 14.1592) (73.7862, 14.0504) (73.5538, 13.9911) knots 0 0 0 1 2 2 2
  line L262 (73.5538, 13.9911) -> (73.4204, 13.9911)
  line L263 (73.4204, 13.9911) -> (73.4204, 17.4168)
  line L264 (73.4204, 17.4168) -> (77.464, 17.4168)
  line L265 (77.464, 17.4168) -> (77.464, 16.265)
  line L266 (77.464, 16.265) -> (74.8688, 16.265)
  line L267 (74.8688, 16.265) -> (74.8688, 15.2517)
  spline S157 degree 2 poles (74.8688, 15.2517) (74.9923, 15.2616) (75.3334, 15.2714) (75.4273, 15.2714) knots 0 0 0 1 2 2 2
  spline S158 degree 2 poles (75.4273, 15.2714) (75.8673, 15.2714) (76.6088, 15.0935) (76.9004, 14.9106) knots 0 0 0 1 2 2 2
  spline S159 degree 2 poles (76.9004, 14.9106) (77.2465, 14.6832) (77.632, 13.9269) (77.632, 13.3831) knots 0 0 0 1 2 2 2
  line L268 (72.5009, -16.1734) -> (71.6754, -16.1734)
  line L269 (71.6754, -16.1734) -> (71.6754, -17.6119)
  line L270 (71.6754, -17.6119) -> (70.1974, -17.6119)
  line L271 (70.1974, -17.6119) -> (70.1974, -16.1734)
  line L272 (70.1974, -16.1734) -> (67.5082, -16.1734)
  line L273 (67.5082, -16.1734) -> (67.5082, -15.0364)
  line L274 (67.5082, -15.0364) -> (70.1479, -11.497)
  line L275 (70.1479, -11.497) -> (71.6754, -11.497)
  line L276 (71.6754, -11.497) -> (71.6754, -15.076)
  line L277 (71.6754, -15.076) -> (72.5009, -15.076)
  line L278 (72.5009, -15.076) -> (72.5009, -16.1734)
  line L279 (70.1974, -15.076) -> (70.1974, -12.9998)
  line L280 (70.1974, -12.9998) -> (68.6501, -15.076)
  line L281 (68.6501, -15.076) -> (70.1974, -15.076)
  spline S160 degree 2 poles (77.7359, -15.5209) (77.7359, -16.4848) (76.5149, -17.7256) (75.4471, -17.7256) knots 0 0 0 1 2 2 2
  spline S161 degree 2 poles (75.4471, -17.7256) (74.9132, -17.7256) (74.0778, -17.4191) (73.7862, -17.1175) knots 0 0 0 1 2 2 2
  spline S162 degree 2 poles (73.7862, -17.1175) (73.4402, -16.7666) (73.0694, -15.6543) (73.0694, -14.8782) knots 0 0 0 1 2 2 2
  spline S163 degree 2 poles (73.0694, -14.8782) (73.0694, -14.0774) (73.4154, -12.8317) (73.806, -12.3522) knots 0 0 0 1 2 2 2
  spline S164 degree 2 poles (73.806, -12.3522) (74.1767, -11.8974) (75.3829, -11.3833) (76.2084, -11.3833) knots 0 0 0 1 2 2 2
  spline S165 degree 2 poles (76.2084, -11.3833) (76.5099, -11.3833) (77.113, -11.4624) (77.2218, -11.4871) knots 0 0 0 1 2 2 2
  line L282 (77.2218, -11.4871) -> (77.2218, -12.6834)
  line L283 (77.2218, -12.6834) -> (77.113, -12.6834)
  spline S166 degree 2 poles (77.113, -12.6834) (77.0043, -12.629) (76.5099, -12.4956) (76.1936, -12.4956) knots 0 0 0 1 2 2 2
  spline S167 degree 2 poles (76.1936, -12.4956) (75.4768, -12.4956) (74.6957, -13.2519) (74.6018, -13.9538) knots 0 0 0 1 2 2 2
  spline S168 degree 2 poles (74.6018, -13.9538) (74.9034, -13.761) (75.5213, -13.5337) (75.9118, -13.5337) knots 0 0 0 1 2 2 2
  spline S169 degree 2 poles (75.9118, -13.5337) (76.243, -13.5337) (76.8214, -13.7116) (77.0438, -13.8797) knots 0 0 0 1 2 2 2
  spline S170 degree 2 poles (77.0438, -13.8797) (77.3602, -14.1219) (77.7359, -14.9079) (77.7359, -15.5209) knots 0 0 0 1 2 2 2
  spline S171 degree 2 poles (75.9513, -16.4403) (76.07, -16.292) (76.1985, -15.946) (76.1985, -15.595) knots 0 0 0 1 2 2 2
  spline S172 degree 2 poles (76.1985, -15.595) (76.1985, -15.2984) (76.0502, -14.9128) (75.9167, -14.7991) knots 0 0 0 1 2 2 2
  spline S173 degree 2 poles (75.9167, -14.7991) (75.7783, -14.6805) (75.4372, -14.5965) (75.2444, -14.5965) knots 0 0 0 1 2 2 2
  spline S174 degree 2 poles (75.2444, -14.5965) (75.0813, -14.5965) (74.7452, -14.6805) (74.5969, -14.7398) knots 0 0 0 1 2 2 2
  spline S175 degree 2 poles (74.5969, -14.7398) (74.5969, -14.7794) (74.587, -14.9672) (74.587, -15.1106) knots 0 0 0 1 2 2 2
  spline S176 degree 2 poles (74.587, -15.1106) (74.587, -15.6395) (74.7699, -16.2772) (74.9132, -16.4403) knots 0 0 0 1 2 2 2
  spline S177 degree 2 poles (74.9132, -16.4403) (75.0171, -16.5738) (75.2939, -16.6875) (75.4422, -16.6875) knots 0 0 0 1 2 2 2
  spline S178 degree 2 poles (75.4422, -16.6875) (75.5658, -16.6875) (75.8525, -16.5639) (75.9513, -16.4403) knots 0 0 0 1 2 2 2
  line L284 (72.5009, -45.0304) -> (71.6754, -45.0304)
  line L285 (71.6754, -45.0304) -> (71.6754, -46.4689)
  line L286 (71.6754, -46.4689) -> (70.1974, -46.4689)
  line L287 (70.1974, -46.4689) -> (70.1974, -45.0304)
  line L288 (70.1974, -45.0304) -> (67.5082, -45.0304)
  line L289 (67.5082, -45.0304) -> (67.5082, -43.8934)
  line L290 (67.5082, -43.8934) -> (70.1479, -40.354)
  line L291 (70.1479, -40.354) -> (71.6754, -40.354)
  line L292 (71.6754, -40.354) -> (71.6754, -43.933)
  line L293 (71.6754, -43.933) -> (72.5009, -43.933)
  line L294 (72.5009, -43.933) -> (72.5009, -45.0304)
  line L295 (70.1974, -43.933) -> (70.1974, -41.8568)
  line L296 (70.1974, -41.8568) -> (68.6501, -43.933)
  line L297 (68.6501, -43.933) -> (70.1974, -43.933)
  line L298 (77.637, -41.5651) -> (75.0319, -46.454)
  line L299 (75.0319, -46.454) -> (73.3314, -46.454)
  line L300 (73.3314, -46.454) -> (76.0551, -41.5058)
  line L301 (76.0551, -41.5058) -> (73.1485, -41.5058)
  line L302 (73.1485, -41.5058) -> (73.1485, -40.354)
  line L303 (73.1485, -40.354) -> (77.637, -40.354)
  line L304 (77.637, -40.354) -> (77.637, -41.5651)
  line L305 (72.5009, -73.8923) -> (71.6754, -73.8923)
  line L306 (71.6754, -73.8923) -> (71.6754, -75.3308)
  line L307 (71.6754, -75.3308) -> (70.1974, -75.3308)
  line L308 (70.1974, -75.3308) -> (70.1974, -73.8923)
  line L309 (70.1974, -73.8923) -> (67.5082, -73.8923)
  line L310 (67.5082, -73.8923) -> (67.5082, -72.7554)
  line L311 (67.5082, -72.7554) -> (70.1479, -69.216)
  line L312 (70.1479, -69.216) -> (71.6754, -69.216)
  line L313 (71.6754, -69.216) -> (71.6754, -72.7949)
  line L314 (71.6754, -72.7949) -> (72.5009, -72.7949)
  line L315 (72.5009, -72.7949) -> (72.5009, -73.8923)
  line L316 (70.1974, -72.7949) -> (70.1974, -70.7187)
  line L317 (70.1974, -70.7187) -> (68.6501, -72.7949)
  line L318 (68.6501, -72.7949) -> (70.1974, -72.7949)
  spline S179 degree 2 poles (77.7556, -73.6204) (77.7556, -74.0109) (77.4294, -74.6882) (77.1179, -74.9353) knots 0 0 0 1 2 2 2
  spline S180 degree 2 poles (77.1179, -74.9353) (76.8065, -75.1825) (75.9118, -75.4593) (75.3334, -75.4593) knots 0 0 0 1 2 2 2
  spline S181 degree 2 poles (75.3334, -75.4593) (74.7155, -75.4593) (73.7911, -75.1776) (73.4945, -74.9353) knots 0 0 0 1 2 2 2
  spline S182 degree 2 poles (73.4945, -74.9353) (73.2029, -74.6931) (72.9261, -74.0357) (72.9261, -73.6699) knots 0 0 0 1 2 2 2
  spline S183 degree 2 poles (72.9261, -73.6699) (72.9261, -73.1459) (73.5044, -72.4489) (74.0531, -72.2165) knots 0 0 0 1 2 2 2
  line L319 (74.0531, -72.2165) -> (74.0531, -72.1918)
  spline S184 degree 2 poles (74.0531, -72.1918) (73.5143, -71.9298) (73.0892, -71.1834) (73.0892, -70.7237) knots 0 0 0 1 2 2 2
  spline S185 degree 2 poles (73.0892, -70.7237) (73.0892, -70.3875) (73.3858, -69.7993) (73.6774, -69.5669) knots 0 0 0 1 2 2 2
  spline S186 degree 2 poles (73.6774, -69.5669) (73.9592, -69.3445) (74.8144, -69.0776) (75.3483, -69.0776) knots 0 0 0 1 2 2 2
  spline S187 degree 2 poles (75.3483, -69.0776) (75.9118, -69.0776) (76.7521, -69.3198) (77.024, -69.5175) knots 0 0 0 1 2 2 2
  spline S188 degree 2 poles (77.024, -69.5175) (77.3008, -69.7152) (77.5974, -70.2887) (77.5974, -70.6199) knots 0 0 0 1 2 2 2
  spline S189 degree 2 poles (77.5974, -70.6199) (77.5974, -71.0549) (77.0932, -71.7519) (76.5742, -71.9941) knots 0 0 0 1 2 2 2
  line L320 (76.5742, -71.9941) -> (76.5742, -72.0139)
  spline S190 degree 2 poles (76.5742, -72.0139) (77.1822, -72.261) (77.7556, -73.0618) (77.7556, -73.6204) knots 0 0 0 1 2 2 2
  spline S191 degree 2 poles (76.243, -73.6847) (76.243, -73.3832) (75.9859, -73.0668) (75.5707, -72.8641) knots 0 0 0 1 2 2 2
  spline S192 degree 2 poles (75.5707, -72.8641) (75.4521, -72.8097) (75.0022, -72.6367) (74.8292, -72.5626) knots 0 0 0 1 2 2 2
  spline S193 degree 2 poles (74.8292, -72.5626) (74.671, -72.7208) (74.4189, -73.1953) (74.4189, -73.4771) knots 0 0 0 1 2 2 2
  spline S194 degree 2 poles (74.4189, -73.4771) (74.4189, -73.9022) (74.9627, -74.4114) (75.4026, -74.4114) knots 0 0 0 1 2 2 2
  spline S195 degree 2 poles (75.4026, -74.4114) (75.5262, -74.4114) (75.8327, -74.3323) (75.9513, -74.2532) knots 0 0 0 1 2 2 2
  spline S196 degree 2 poles (75.9513, -74.2532) (76.0848, -74.1592) (76.243, -73.9022) (76.243, -73.6847) knots 0 0 0 1 2 2 2
  spline S197 degree 2 poles (76.1095, -70.7978) (76.1095, -70.4864) (75.6992, -70.1156) (75.3483, -70.1156) knots 0 0 0 1 2 2 2
  spline S198 degree 2 poles (75.3483, -70.1156) (75.0121, -70.1156) (74.6018, -70.4518) (74.6018, -70.699) knots 0 0 0 1 2 2 2
  spline S199 degree 2 poles (74.6018, -70.699) (74.6018, -70.9412) (74.849, -71.2427) (75.111, -71.3663) knots 0 0 0 1 2 2 2
  spline S200 degree 2 poles (75.111, -71.3663) (75.2247, -71.4256) (75.541, -71.5492) (75.803, -71.6481) knots 0 0 0 1 2 2 2
  spline S201 degree 2 poles (75.803, -71.6481) (75.9612, -71.4404) (76.1095, -71.0499) (76.1095, -70.7978) knots 0 0 0 1 2 2 2
  point P0 (0, 0)
  constraints: 100 end point, 20 point on line, 12 horizontal, 9 vertical, 3 collinear, 3 perpendicular, 1 midpoint, 24 other
extrude "Extrusión13" cut sketch "Boceto13" against normal blind 1.5 contours L111 L112 L113 L0 | L0 L113 L114 L115 L116 L117 L111 | L202 L203 L204 L2 L207 L208 | L2 L208 L209 L207 L204 L205 L206 L196 L197 L198 L199 L200 L201 L202 | S18 S19 S0 S1 S2 L103 L104 S3 S4 S5 S6 S7 L105 L106 L0 | L0 L106 L107 S8 S9 S10 S11 S12 S13 L108 L109 S14 S15 S16 S17 L110 S18 | S51 S40 S41 S42 S43 S44 L5 | L5 S44 L126 S45 S46 S47 S48 S49 S50 L127 S51 | L121 L122 S28 S29 S30 S31 S32 S33 L123 L124 S34 S35 S36 S37 L125 S38 L5 | L5 S38 S39 S20 S21 S22 L118 L119 S23 S24 S25 S26 S27 L120 L121 | L224 L225 L226 L6 L229 L230 | L6 L230 L231 L229 L226 L227 L228 L218 L219 L220 L221 L222 L223 L224 | S145 S146 S127 S128 S129 L210 L211 S130 S131 S132 S133 S134 L212 L213 L2 | L2 L213 L214 S135 S136 S137 S138 S139 S140 L215 L216 S141 S142 S143 S144 L217 S145 | L240 L241 L242 L232 L233 L234 L235 L236 L237 L238 L6 L244 L245 L243 | L6 L243 L244 L238 L239 L240 | L131 L132 S71 S72 S73 S74 S75 S76 L133 L134 S77 S78 S79 S80 L135 S81 L8 | L8 S81 S82 S63 S64 S65 L128 L129 S66 S67 S68 S69 S70 L130 L131 | L252 L253 L254 L9 L257 L258 | L9 L258 L259 L257 L254 L255 L256 L246 L247 L248 L249 L250 L251 L252 | S83 S84 S85 L136 L137 S86 S87 S88 S89 S90 S91 L8 | L8 S91 S92 S93 S94 S95 S83 | S159 S147 S148 S149 L260 L261 S150 S151 S152 S153 S154 S155 S156 L262 L263 L9 | L9 L263 L264 L265 L266 L267 S157 S158 S159 | L144 L145 L146 L11 L149 L150 | L11 L150 L151 L149 L146 L147 L148 L138 L139 L140 L141 L142 L143 L144 | L274 L275 L276 L12 L279 L280 | L12 L280 L281 L279 L276 L277 L278 L268 L269 L270 L271 L272 L273 L274 | S104 S105 S106 S107 L11 S113 S114 S115 | L11 S112 S113 S108 S109 S110 S111 | S170 S160 S161 S162 S163 L12 | L12 S163 S164 S165 L282 L283 S166 S167 S168 S169 S170 | L158 L159 L160 L14 L163 L164 | L14 L164 L165 L163 L160 L161 L162 L152 L153 L154 L155 L156 L157 L158 | L173 L174 L175 L166 L167 L168 L169 L14 | L14 L169 L170 L171 S116 S117 L172 L173 | L298 L299 L300 L15 | L15 L300 L301 L302 L303 L304 L298 | L290 L291 L292 L15 L295 L296 | L15 L296 L297 L295 L292 L293 L294 L284 L285 L286 L287 L288 L289 L290 | L182 L183 L184 L18 L187 L188 | L18 L188 L189 L187 L184 L185 L186 L176 L177 L178 L179 L180 L181 L182 | S125 S126 L194 L195 L190 L191 S118 S119 L18 | L18 S119 S120 S121 S122 L192 L193 S123 S124 S125 | S190 S179 S180 S181 S182 S183 L19 | L19 S183 L319 S184 S185 S186 S187 S188 S189 L320 S190 | L311 L312 L313 L19 L316 L317 | L19 L317 L318 L316 L313 L314 L315 L305 L306 L307 L308 L309 L310 L311
